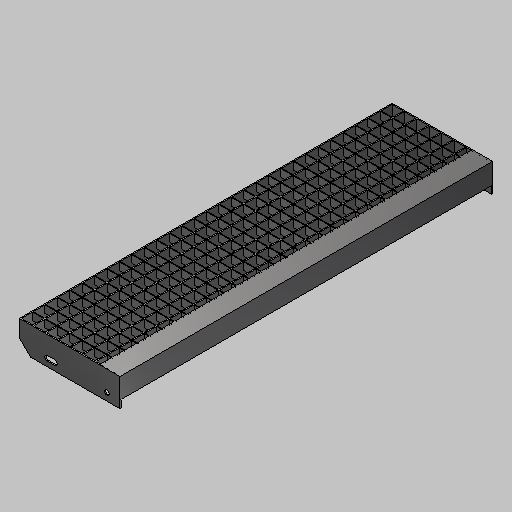
# Autodesk Inventor part: Tread
Saved by Autodesk Inventor 2026.2 (Build 302298000, 298)
## iProperties
Created: 2015-03-25
Part Number: Tread
Material: Steel, Galvanized
Document SubType Name: Modeling
Designer: m_crauwels
Density: 7.85 g/cm^3
Appearance: Galvanized
Mass: 7101.07 g
Surface Area: 7597.27 cm^2
Volume: 904.595 cm^3
d0: 500,000 mm
d1: 270.000 mm
d2: 75.000 mm
d3: 30.000 mm
d4: 30.000 mm
d5: 3.000 mm
d6: 0.00 deg
d7: 35.000 mm
d8: 55.000 mm
d9: 13.000 mm
d10: 20.000 mm
d11: 13.000 mm
d12: 150.000 mm
d14: 0.00 deg
d15: 2.000 mm
d16: 55.000 mm
d17: 2.000 mm
d18: 55.000 mm
d19: 30.000 mm
d21: 0.00 deg
d22: 3.000 mm
d23: 30.000 mm
d25: 0.00 deg
d26: 7.000 ul
d28: 33.330 mm
d29: 20.000 mm
d30: 2.000 mm
StairsWidth: 1000,000 mm
Author: m_crauwels
Autodesk Inventor part; units mm, degrees
ref_plane "YZ Plane" through (0, 0, 0) normal (1, 0, 0) x (0, 1, 0)
ref_plane "XY Plane" through (0, 0, 0) normal (0, 0, 1) x (1, 0, 0)
ref_plane "Work Plane1" through (0, 500, 0) normal (0, 1, 0) x (-1, 0, 0)
sketch "Sketch1" plane through (0, 500, 0) normal (0, 1, 0) x (-1, 0, 0)
  line L0 (0, 0) -> (270, 0)
  line L1 (270, 0) -> (270, -75)
  line L2 (270, -75) -> (0, -75)
  line L3 (0, -75) -> (0, 0)
  line L4 (270, -45) -> (240, -75)
  dimension "d1" = 270
  dimension "d2" = 75
  dimension "d3" = 30
  dimension "d4" = 30
  constraints: 10 end point, 2 parallel, 2 point on line, 1 horizontal, 1 perpendicular
  measures "d1" distance of L1.end L2.end
  measures "d2" distance of L0.end L1.end
  measures "d3" distance of L1.end L4.start
  measures "d4" distance of L4.end L1.end
extrude "Extrusion1" add sketch "Sketch1" against normal blind 3 contours L0 L1 L4 L2 L3
sketch "Sketch2" plane through (0, 497, 0) normal (0, -1, 0) x (1, 0, 0)
  line L0 (0, -75) -> (0, 0) projected
  line L1 (0, 0) -> (-270, 0) projected
  line L2 (-240, -75) -> (0, -75) projected
  line L3 (0, -55) -> (-35, -55) construction
  line L4 (-35, -55) -> (-35, 0) construction
  circle A0 centre (-35, -55) radius 6.5
  line L5 (-175, -55) -> (-195, -55) construction
  line L6 (-175, -48.5) -> (-195, -48.5)
  line L7 (-195, -61.5) -> (-175, -61.5)
  arc A1 (-175, -61.5) -> (-175, -48.5) centre (-175, -55) ccw
  arc A2 (-195, -48.5) -> (-195, -61.5) centre (-195, -55) ccw
  point P0 (-185, -55)
  dimension "d31" = 3
  dimension "d7" = 35
  dimension "d8" = 55
  dimension "d9" = 13
  dimension "d10" = 20
  dimension "d11" = 13
  dimension "d12" = 150
  constraints: 12 end point, 4 point on circle, 4 tangent, 3 centre point, 3 parallel, 2 point on line, 1 coincident, 1 collinear, 1 midpoint, 1 perpendicular
  measures "d7" distance of L3.start L3.end
  measures "d8" distance of L3.end L4.end
  measures "d9" diameter of A0
  measures "d10" distance of L5.start L5.end
  measures "d11" diameter of A2
  measures "d12" distance from line of point (-185, -55) L4
extrude "Extrusion2" cut sketch "Sketch2" against normal through all
mirror "Mirror1" about plane through (0, 0, 0) normal (0, 1, 0) of "Extrusion1", "Extrusion2"
sketch "Sketch3" plane through (0, 497, 0) normal (0, -1, 0) x (1, 0, 0)
  line L0 (0, -75) -> (0, 0) projected
  line L1 (0, 0) -> (-270, 0) projected
  line L2 (-55, -30) -> (-55, 0)
  line L3 (-55, -30) -> (-53, -30)
  line L4 (-53, -30) -> (-53, -2)
  line L5 (-53, -2) -> (-2, -2)
  line L6 (-2, -2) -> (-2, -55)
  line L7 (-2, -55) -> (0, -55)
  dimension "d15" = 2
  dimension "d16" = 55
  dimension "d17" = 2
  dimension "d18" = 55
  dimension "d19" = 30
  constraints: 12 end point, 4 perpendicular, 3 parallel, 2 point on line
  measures "d15" distance of L2.start L3.end
  measures "d16" distance of L0.end L7.end
  measures "d17" distance between parallel lines of L1 L5
  measures "d18" distance between parallel lines of L2 L0
  measures "d19" distance of L2.start L2.end
extrude "Extrusion3" add sketch "Sketch3" along normal up to surface (994 mm away)
sketch "Sketch4" plane through (0, 497, 0) normal (0, -1, 0) x (1, 0, 0)
  line L0 (-270, 0) -> (-267, 0)
  line L1 (-267, 0) -> (-267, -30)
  line L2 (-267, -30) -> (-270, -30)
  line L3 (-270, -30) -> (-270, 0)
  point P0 (0, 0)
  dimension "d22" = 3
  dimension "d23" = 30
  constraints: 8 end point, 2 parallel, 1 horizontal, 1 perpendicular
  measures "d22" distance of L1.end L2.end
  measures "d23" distance of L0.end L1.end
extrude "Extrusion4" add sketch "Sketch4" along normal up to surface (994 mm away)
pattern_linear "Rectangular Pattern1" count 7 spacing 33.33 along (1, 0, 0) of "Extrusion4"
sketch "Sketch5" plane through (-267, 497, 0) normal (1, 0, 0) x (0, 0, -1)
  line L0 (0, 0) -> (0, -994) projected
  line L1 (0, -498) -> (20, -498)
  line L2 (20, -498) -> (20, -496)
  line L3 (20, -496) -> (0, -496)
  line L4 (0, -496) -> (0, -498)
  point P0 (0, -497)
  point P1 (0, -497)
  dimension "d29" = 20
  dimension "d30" = 2
  constraints: 8 end point, 2 midpoint, 2 parallel, 1 horizontal, 1 perpendicular
  measures "d29" distance of L3.end L2.end
  measures "d30" distance of L2.end L1.end
extrude "Extrusion5" add sketch "Sketch5" along normal up to surface (212 mm away)
pattern_linear "Rectangular Pattern2" count 29 spacing 33.33 along (0, -1, 0) of "Extrusion5" first direction both ways yes
equation "\"d17\" = d15"
equation "\"d18\" = d16"
equation "\"d0\" = 0.5 * StairsWidth"
equation "\"StairsWidth\" = 1000"
body "Solid1"
